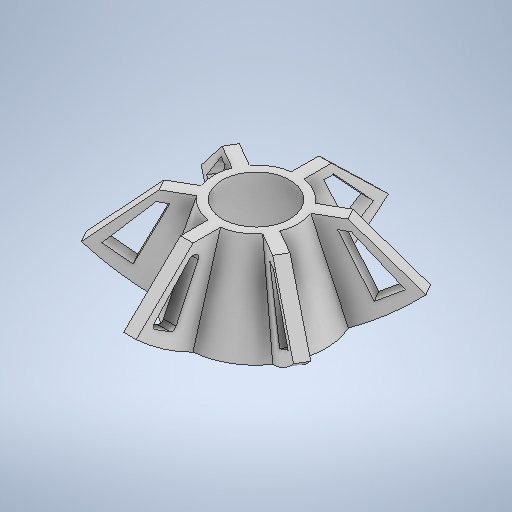
# Autodesk Inventor part: Internal Structure
Saved by Autodesk Inventor 2026.2 (Build 302298000, 298)
## iProperties
Created: 2026-01-18
Part Number: Internal Structure
Material: Generic
Document SubType Name: Modeling
Designer: daryu
Density: 1 g/cm^3
Appearance: Default
Author: daryu
Autodesk Inventor part; units mm, degrees
ref_plane "YZ Plane" through (0, 0, 0) normal (1, 0, 0) x (0, 1, 0)
ref_plane "XZ Plane" through (0, 0, 0) normal (0, 1, 0) x (-1, 0, 0)
ref_plane "XY Plane" through (0, 0, 0) normal (0, 0, 1) x (1, 0, 0)
sketch "Sketch1" plane through (0, 0, 0) normal (1, 0, 0) x (0, 1, 0)
  line L0 (0, 14.7987) -> (0, -14.7987)
  line L1 (20.2387, -8.912) -> (20.2387, 8.912)
  line L2 (0, 14.7987) -> (20.2387, 8.912)
  line L3 (20.2387, 8.912) -> (23.2652, 8.0317)
  line L4 (23.2652, 8.0317) -> (23.2652, 10.0317)
  line L5 (23.2652, 10.0317) -> (0.8483, 16.552)
  arc A0 (10.1758, 29.9776) -> (0, 14.7987) centre (53.1668, -9.8435) ccw
  line L6 (0, 0) -> (4.1623, 0)
  dimension "d0" = 2
  dimension "d1" = 23.3459
  dimension "d2" = 58.5999
  dimension "d3" = 29.5974
  dimension "d4" = 20.2387
  dimension "d5" = 17.8241
  dimension "d6" = 1.7533
  constraints: 14 end point, 3 point on circle, 1 centre point, 1 coincident, 1 horizontal, 1 midpoint, 1 parallel, 1 perpendicular, 1 point on line, 1 vertical
  measures "d0" distance of L3.end L4.end
  measures "d1" distance of L4.end L5.end
  measures "d2" radius of A0
  measures "d3" distance of L0.start L0.end
  measures "d4" horizontal distance of L0.start L1.end
  measures "d5" distance of L1.start L1.end
  measures "d6" vertical distance of L0.start L5.end
revolve "Revolution1" add sketch "Sketch1" angle 360 about axis through (0, 0, 0) along (0, 1, 0)
sketch "Sketch2" plane through (0, 0, 0) normal (1, 0, 0) x (0, 1, 0)
  arc A0 (10.1596, 29.9776) -> (0.8483, 16.552) centre (53.1862, -9.8051) ccw
  line L0 (0.8483, 16.552) -> (23.2652, 10.0317)
  line L1 (23.2652, 9.4492) -> (23.2652, 16.4492)
  line L2 (10.1596, 29.9776) -> (23.2652, 16.4492)
  line L3 (0.8483, -16.552) -> (23.2652, -10.0317) projected
  line L4 (0.8483, 16.552) -> (23.2652, 10.0317) projected
  line L5 (10.5533, 26.4347) -> (20.7474, 17.0064)
  line L6 (7.1516, 20.973) -> (10.5533, 26.4347)
  line L7 (7.1516, 20.973) -> (20.7474, 14.6029)
  line L8 (20.7474, 17.0064) -> (20.7474, 14.6029)
  line L9 (23.2652, 9.4492) -> (0.7694, 16.1344)
  line L10 (0.7694, 16.1344) -> (0.8483, 16.552)
  point P0 (0, 0)
  dimension "d8" = 18.8355
  dimension "d9" = 22.4169
  dimension "d10" = 7
  dimension "d11" = 58.5999
  dimension "d12" = 23.3459
  dimension "d15" = 13.4256
  constraints: 18 end point, 2 point on circle, 2 vertical, 1 centre point
  measures "d8" distance of L2.start L1.end
  measures "d9" horizontal distance of L0.end L0.start
  measures "d10" distance of L1.start L1.end
  measures "d11" radius of A0
  measures "d12" distance of L0.end L0.start
  measures "d15" vertical distance of L4.start L2.start
extrude "Extrusion1" add sketch "Sketch2" along normal mid plane 3
fillet "Fillet1" radius 1 4 edges at (0, 10.5533, 26.4347) (0, 7.1516, 20.973) (0, 20.7474, 17.0064) (0, 20.7474, 14.6029)
pattern_circular "Circular Pattern1" count 6 over 360 about axis through (0, 11.6326, 0) along (0, 1, 0) of "Extrusion1"
body "Solid1"
